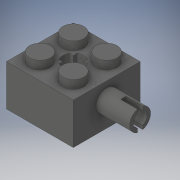
# Autodesk Inventor part: 2x2 tall things sticking out
Saved by Autodesk Inventor 2017 (Build 210142000, 142)
## iProperties
Created: 2018-05-17
Part Number: 2x2 tall things sticking out
Material: ABS Plastic
Document SubType Name: Modeling
Designer: Kyle
Density: 1.06 g/cm^3
Appearance: Gray
Author: Kyle
Autodesk Inventor part; units mm, degrees
ref_plane "YZ Plane" through (0, 0, 0) normal (1, 0, 0) x (0, 1, 0)
ref_plane "XZ Plane" through (0, 0, 0) normal (0, 1, 0) x (-1, 0, 0)
ref_plane "XY Plane" through (0, 0, 0) normal (0, 0, 1) x (1, 0, 0)
sketch "Sketch1" plane through (0, 0, 0) normal (0, 1, 0) x (-1, 0, 0)
  line L0 (0, 0) -> (15.5956, 0)
  line L1 (15.5956, 0) -> (15.5956, -15.5956)
  line L2 (15.5956, -15.5956) -> (0, -15.5956)
  line L3 (0, -15.5956) -> (0, 0)
  dimension "d0" = 15.5956
  dimension "d8" = 15.5956
  constraints: 8 end point, 2 parallel, 1 horizontal, 1 perpendicular
  measures "d0" distance of L1.end L2.end
  measures "d8" distance of L0.end L1.end
extrude "Extrusion1" add sketch "Sketch1" along normal blind 9.6088
sketch "Sketch2" plane through (0, 9.6088, 0) normal (0, 1, 0) x (1, 0, 0)
  line L0 (0, 0) -> (-3.8989, 0) construction
  line L1 (-3.8989, 0) -> (-3.8989, 3.8989) construction
  line L2 (-3.8989, 3.8989) -> (0, 3.8989) construction
  line L3 (0, 3.8989) -> (0, 0) construction
  circle A0 centre (-3.8989, 3.8989) radius 2.4498
  dimension "d11" = 3.8989
  dimension "d12" = 3.8989
  dimension "d13" = 4.8997
  constraints: 8 end point, 2 parallel, 1 centre point, 1 coincident, 1 horizontal, 1 perpendicular
  measures "d11" distance of L1.end L2.end
  measures "d12" distance of L0.end L1.end
  measures "d13" diameter of A0
extrude "Extrusion2" add sketch "Sketch2" along normal blind 1.9837
pattern_linear "Rectangular Pattern1" count 2 spacing 7.7978 along (0, 0, -1) count 2 spacing 7.7978 along (-1, 0, 0) of "Extrusion2"
shell "Shell1" thickness 1.4732 removed faces 1 at (-5.1985, 0, -5.1985)
sketch "Sketch3" plane through (-14.1224, 8.1356, -1.4732) normal (0, -1, 0) x (1, 0, 0)
  circle A0 centre (2.4257, -2.4257) radius 2.4498 construction
  circle A1 centre (10.2235, -10.2235) radius 2.4498 construction
  line L0 (2.4257, -2.4257) -> (10.2235, -10.2235) construction
  circle A2 centre (6.3246, -6.3246) radius 3.064
  circle A3 centre (6.3246, -6.3246) radius 2.4498
  point P0 (14.1224, 1.4732)
  dimension "d23" = 4.8997
  constraints: 2 centre point, 2 end point, 1 coincident, 1 midpoint
  measures "d23" diameter of A3
extrude "Extrusion3" add sketch "Sketch3" along normal up to surface (8.1356 mm away)
sketch "Sketch4" plane through (0, 9.6088, 0) normal (0, 1, 0) x (1, 0, 0)
  circle A0 centre (-7.7978, 7.7978) radius 2.4498 construction
  circle A1 centre (-7.7978, 7.7978) radius 2.4498 construction
  line L0 (-9.0227, 5.6762) -> (-6.5729, 5.6762) construction
  line L1 (-6.5729, 5.6762) -> (-6.5729, 9.9194) construction
  line L2 (-6.5729, 9.9194) -> (-9.0227, 9.9194) construction
  line L3 (-9.0227, 9.9194) -> (-9.0227, 5.6762) construction
  line L4 (-9.0227, 5.6762) -> (-6.5729, 9.9194) construction
  line L5 (-6.5729, 5.6762) -> (-9.0227, 9.9194) construction
  line L6 (-9.9194, 9.0227) -> (-5.6762, 9.0227) construction
  line L7 (-5.6762, 9.0227) -> (-5.6762, 6.5729) construction
  line L8 (-5.6762, 6.5729) -> (-9.9194, 6.5729) construction
  line L9 (-9.9194, 6.5729) -> (-9.9194, 9.0227) construction
  line L10 (-9.9194, 9.0227) -> (-5.6762, 6.5729) construction
  line L11 (-5.6762, 9.0227) -> (-9.9194, 6.5729) construction
  line L12 (-9.0227, 9.0227) -> (-9.0227, 9.9194)
  line L13 (-6.5729, 9.9194) -> (-6.5729, 9.0227)
  line L14 (-6.5729, 9.0227) -> (-5.6762, 9.0227)
  line L15 (-5.6762, 6.5729) -> (-6.5729, 6.5729)
  line L16 (-6.5729, 6.5729) -> (-6.5729, 5.6762)
  line L17 (-9.0227, 5.6762) -> (-9.0227, 6.5729)
  line L18 (-9.0227, 6.5729) -> (-9.9194, 6.5729)
  line L19 (-9.9194, 9.0227) -> (-9.0227, 9.0227)
  arc A2 (-9.9194, 9.0227) -> (-9.9194, 6.5729) centre (-7.7978, 7.7978) ccw
  arc A3 (-6.5729, 9.9194) -> (-9.0227, 9.9194) centre (-7.7978, 7.7978) ccw
  arc A4 (-5.6762, 6.5729) -> (-5.6762, 9.0227) centre (-7.7978, 7.7978) ccw
  arc A5 (-9.0227, 5.6762) -> (-6.5729, 5.6762) centre (-7.7978, 7.7978) ccw
  point P0 (0, 0)
  dimension "d26" = 2.4498
  dimension "d27" = 2.4498
  constraints: 40 end point, 10 point on circle, 8 point on line, 4 centre point, 4 midpoint, 4 parallel, 4 perpendicular, 3 collinear, 2 horizontal
  measures "d26" distance of L2.end L1.end
  measures "d27" distance of L6.end L7.end
extrude "Extrusion4" cut sketch "Sketch4" against normal through all
sketch "Sketch5" plane through (0, 0, 0) normal (1, 0, 0) x (0, 0, -1)
  line L0 (0, 9.6088) -> (7.7978, 9.6088) construction
  line L1 (7.7978, 9.6088) -> (7.7978, 5.7099) construction
  line L2 (7.7978, 5.7099) -> (0, 5.7099) construction
  line L3 (0, 5.7099) -> (0, 9.6088) construction
  circle A0 centre (7.7978, 5.7099) radius 2.4498
  point P0 (0, 0)
  dimension "d30" = 7.7978
  dimension "d31" = 3.8989
  dimension "d32" = 4.8997
  constraints: 8 end point, 2 parallel, 1 centre point, 1 coincident, 1 horizontal, 1 perpendicular
  measures "d30" distance of L1.end L2.end
  measures "d31" distance of L0.end L1.end
  measures "d32" diameter of A0
extrude "Extrusion5" add sketch "Sketch5" along normal blind 7.7978
sketch "Sketch6" plane through (7.7978, 5.7099, -7.7978) normal (1, 0, 0) x (0, 0, -1)
  circle A0 centre (0, 0) radius 2.4498 construction
  circle A1 centre (0, 0) radius 1.618
  point P0 (-7.7978, -5.7099)
  dimension "d35" = 3.236
  constraints: 1 centre point, 1 coincident
  measures "d35" diameter of A1
extrude "Extrusion6" cut sketch "Sketch6" against normal blind 7.7978
sketch "Sketch7" plane through (-6.5729, 8.1356, -9.0227) normal (0, -1, 0) x (1, 0, 0)
  line L0 (-2.4498, 2.4498) -> (-2.4498, 3.3465) construction
  arc A0 (-2.4498, 3.3465) -> (-3.3465, 2.4498) centre (-1.2249, 1.2249) ccw construction
  line L1 (-3.3465, 2.4498) -> (-2.4498, 2.4498) construction
  line L2 (0, 2.4498) -> (0.8967, 2.4498) construction
  arc A1 (0.8967, 2.4498) -> (0, 3.3465) centre (-1.2249, 1.2249) ccw construction
  line L3 (0, 3.3465) -> (0, 2.4498) construction
  line L4 (0.8967, 0) -> (0, 0) construction
  line L5 (0, 0) -> (0, -0.8967) construction
  arc A2 (0, -0.8967) -> (0.8967, 0) centre (-1.2249, 1.2249) ccw construction
  line L6 (-2.4498, -0.8967) -> (-2.4498, 0) construction
  line L7 (-2.4498, 0) -> (-3.3465, 0) construction
  arc A3 (-3.3465, 0) -> (-2.4498, -0.8967) centre (-1.2249, 1.2249) ccw construction
  arc A4 (-2.4498, 3.3465) -> (-3.3465, 2.4498) centre (-1.2249, 1.2249) ccw
  arc A5 (0.8967, 0) -> (0.8967, 2.4498) centre (-1.2249, 1.2249) ccw projected
  arc A6 (0.8967, 2.4498) -> (0, 3.3465) centre (-1.2249, 1.2249) ccw
  arc A7 (-2.4498, -0.8967) -> (0, -0.8967) centre (-1.2249, 1.2249) ccw projected
  arc A8 (0, -0.8967) -> (0.8967, 0) centre (-1.2249, 1.2249) ccw
  arc A9 (-3.3465, 0) -> (-2.4498, -0.8967) centre (-1.2249, 1.2249) ccw
  line L8 (-2.4498, 3.3465) -> (-2.4498, 2.4498)
  line L9 (-2.4498, 2.4498) -> (-3.3465, 2.4498) projected
  line L10 (-2.4498, 2.4498) -> (-3.3465, 2.4498)
  line L11 (0, 2.4498) -> (0, 3.3465) projected
  line L12 (0, 3.3465) -> (0, 2.4498)
  line L13 (0, 2.4498) -> (0.8967, 2.4498)
  line L14 (0, 0) -> (0.8967, 0) projected
  line L15 (0.8967, 0) -> (0, 0)
  line L16 (0, 0) -> (0, -0.8967)
  line L17 (-2.4498, 0) -> (-2.4498, -0.8967) projected
  line L18 (-2.4498, -0.8967) -> (-2.4498, 0)
  arc A10 (-3.3465, 2.4498) -> (-3.3465, 0) centre (-1.2249, 1.2249) ccw projected
  line L19 (-2.4498, 0) -> (-3.3465, 0)
  point P0 (6.5729, 9.0227)
  constraints: 16 end point, 8 point on circle, 4 centre point, 3 vertical, 2 collinear, 2 perpendicular, 1 concentric
extrude "Extrusion7" add sketch "Sketch7" along normal up to surface (8.1356 mm away)
sketch "Sketch8" plane through (-7.7978, 0, -7.7978) normal (0, -1, 0) x (1, 0, 0)
  arc A0 (2.1216, -1.2249) -> (2.1216, 1.2249) centre (0, 0) ccw construction
  line L0 (2.1216, -1.2249) -> (1.2249, -1.2249) construction
  line L1 (1.2249, -1.2249) -> (1.2249, -2.1216) construction
  arc A1 (-1.2249, -2.1216) -> (1.2249, -2.1216) centre (0, 0) ccw construction
  line L2 (-1.2249, -2.1216) -> (-1.2249, -1.2249) construction
  line L3 (-1.2249, -1.2249) -> (-2.1216, -1.2249) construction
  arc A2 (-2.1216, 1.2249) -> (-2.1216, -1.2249) centre (0, 0) ccw construction
  line L4 (-2.1216, 1.2249) -> (-1.2249, 1.2249) construction
  line L5 (-1.2249, 1.2249) -> (-1.2249, 2.1216) construction
  arc A3 (1.2249, 2.1216) -> (-1.2249, 2.1216) centre (0, 0) ccw construction
  line L6 (1.2249, 2.1216) -> (1.2249, 1.2249) construction
  line L7 (1.2249, 1.2249) -> (2.1216, 1.2249) construction
  circle A4 centre (0, 0) radius 3.064 construction
  circle A5 centre (0, 0) radius 2.4498
  point P0 (7.7978, 7.7978)
  constraints: 1 centre point, 1 coincident
extrude "Extrusion8" cut sketch "Sketch8" against normal blind 1.618
ref_plane "Work Plane1" through (0, 8.1598, -7.7978) normal (0, 1, 0) x (-1, 0, 0)
sketch "Sketch9" plane through (0, 8.1598, -7.7978) normal (0, 1, 0) x (-1, 0, 0)
  line L0 (-7.7978, 2.4498) -> (-7.7978, -2.4498) construction
  line L1 (-7.7978, 0) -> (-7.7978, 0.6125) construction
  line L2 (-7.7978, 0) -> (-7.1853, 0) construction
  line L3 (-7.7978, 0.6125) -> (-3.8989, 0.6125)
  line L4 (-3.8989, 0.6125) -> (-3.8989, -0.6125)
  line L5 (-3.8989, -0.6125) -> (-7.7978, -0.6125)
  line L6 (-7.7978, -0.6125) -> (-7.7978, 0.6125)
  point P0 (0, 7.7978)
  dimension "d42" = 0.6125
  dimension "d43" = 90
  dimension "d44" = 3.8989
  dimension "d45" = 1.2249
  constraints: 12 end point, 2 horizontal, 2 parallel, 2 perpendicular, 1 collinear, 1 midpoint
  measures "d42" distance of L1.start L1.end
  measures "d43" angle of L2 L1
  measures "d44" distance of L4.end L5.end
  measures "d45" distance of L3.end L4.end
extrude "Extrusion9" cut sketch "Sketch9" against normal through all
equation "\"d0\" = 2 * d1"
equation "\"d8\" = 2 * d1"
equation "\"d9\" = d3"
equation "\"d11\" = 0.5 * d1"
equation "\"d12\" = 0.5 * d1"
equation "\"d13\" = d4"
equation "\"d14\" = d5"
equation "\"d18\" = d1"
equation "\"d21\" = d1"
equation "\"d22\" = d6"
equation "\"d23\" = d4"
equation "\"d24\" = d5"
equation "\"d26\" = 0.5 * d4"
equation "\"d27\" = 0.5 * d4"
equation "\"d28\" = d5"
equation "\"d30\" = d1"
equation "\"d31\" = 0.5 * d1"
equation "\"d32\" = d4"
equation "\"d33\" = d1"
equation "\"d35\" = d2"
equation "\"d36\" = d1"
equation "\"d40\" = 0.5 * d2"
equation "\"d42\" = 0.125 * d4"
equation "\"d44\" = 0.5 * d1"
equation "\"d45\" = 0.25 * d4"
equation "\"d46\" = 0.5 * d2"
equation "\"d1\" = 7.7978"
equation "\"d2\" = 3.23596"
equation "\"d3\" = 9.60882"
equation "\"d4\" = 4.89966"
equation "\"d5\" = 1.98374"
equation "\"d6\" = 1.4732"
equation "\"d7\" = 1.23952"
body "Solid1"
